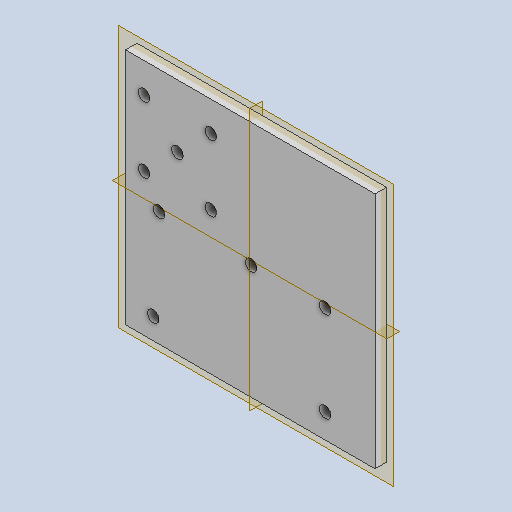
# Autodesk Inventor part: Крыло(подвижная часть)
Saved by Autodesk Inventor 2023.2 (Build 272271030, 271C)
## iProperties
Created: 2024-03-20
Part Number: Крыло(подвижная часть)
Material: Типовые
Document SubType Name: Modeling
Designer: I9232
Density: 1 g/cm^3
Appearance: По умолчанию
Author: I9232
Autodesk Inventor part; units mm, degrees
sketch "Эскиз1" plane through (0, 0, 0) normal (0, 0, 1) x (1, 0, 0)
  line L0 (-43.5, -41.5) -> (43.5, -41.5)
  line L1 (43.5, -41.5) -> (43.5, 41.5)
  line L2 (43.5, 41.5) -> (-43.5, 41.5)
  line L3 (-43.5, 41.5) -> (-43.5, -41.5)
  line L4 (-43.5, -41.5) -> (43.5, 41.5) construction
  line L5 (43.5, -41.5) -> (-43.5, 41.5) construction
  point P0 (0, 0)
  dimension "d0" = 87
  dimension "d1" = 83
  constraints: 12 end point, 2 midpoint, 2 parallel, 1 horizontal, 1 perpendicular
  measures "d0" distance of L1.end L2.end
  measures "d1" distance of L0.end L1.end
extrude "Выдавливание1" add sketch "Эскиз1" along normal mid plane 4
sketch "Эскиз2" plane through (0, 0, 2) normal (0, 0, 1) x (1, 0, 0)
  circle A0 centre (-33.8217, -34.089) radius 2
  circle A1 centre (-31.8217, -1.5) radius 2
  circle A2 centre (-37.0131, 8.089) radius 2
  circle A3 centre (-13.7428, 8.089) radius 2
  circle A4 centre (0.3071, -1.6211) radius 2
  circle A5 centre (-25.378, 19.589) radius 2
  circle A6 centre (-37.0131, 31.089) radius 2
  circle A7 centre (-13.7428, 31.089) radius 2
  circle A8 centre (26.084, -1.6211) radius 2
  circle A9 centre (26.084, -33.0251) radius 2
  point P0 (0, 0)
  constraints: 10 centre point
extrude "Выдавливание2" cut sketch "Эскиз2" against normal up to surface (4 mm away)
